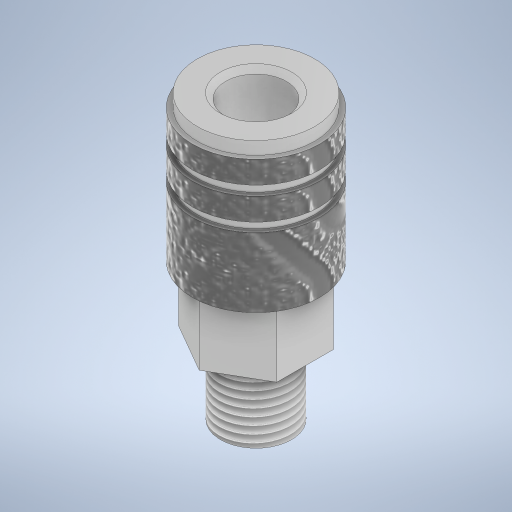
# Autodesk Inventor part: AcopleHembra
Saved by Autodesk Inventor 2024 (Build 280153000, 153)
## iProperties
Created: 2024-04-30
Part Number: AcopleHembra
Material: Genérico
Document SubType Name: Modeling
Designer: alexa
Density: 1 g/cm^3
Appearance: Valor por defecto
Author: alexa
Autodesk Inventor part; units mm, degrees
ref_plane "YZ Plane" through (0, 0, 0) normal (1, 0, 0) x (0, 1, 0)
ref_plane "XZ Plane" through (0, 0, 0) normal (0, 1, 0) x (-1, 0, 0)
ref_plane "XY Plane" through (0, 0, 0) normal (0, 0, 1) x (1, 0, 0)
sketch "Sketch1" plane through (0, 0, 0) normal (0, 1, 0) x (-1, 0, 0)
  circle A0 centre (0, 0) radius 6.65
  dimension "d0" = 13.3
  constraints: 1 centre point, 1 coincident
  measures "d0" diameter of A0
extrude "Extrusion1" add sketch "Sketch1" along normal blind 13.3
sketch "Sketch2" plane through (0, 13.3, 0) normal (0, 1, 0) x (1, 0, 0)
  line L0 (0, 10.65) -> (9.2232, 5.325)
  line L1 (9.2232, 5.325) -> (9.2232, -5.325)
  line L2 (9.2232, -5.325) -> (0, -10.65)
  line L3 (0, -10.65) -> (-9.2232, -5.325)
  line L4 (-9.2232, -5.325) -> (-9.2232, 5.325)
  line L5 (-9.2232, 5.325) -> (0, 10.65)
  point P0 (0, 0)
  point P1 (0, 0)
  constraints: 12 end point, 13 other
extrude "Extrusion2" add sketch "Sketch2" along normal blind 12.4
sketch "Sketch3" plane through (0, 25.7, 0) normal (0, 1, 0) x (1, 0, 0)
  circle A0 centre (0, 0) radius 11.9
  dimension "d6" = 23.8
  constraints: 1 centre point, 1 coincident
  measures "d6" diameter of A0
extrude "Extrusion3" add sketch "Sketch3" along normal blind 13
sketch "Sketch4" plane through (0, 38.7, 0) normal (0, 1, 0) x (1, 0, 0)
  circle A0 centre (0, 0) radius 11
  dimension "d9" = 22
  constraints: 1 centre point, 1 coincident
  measures "d9" diameter of A0
extrude "Extrusion4" add sketch "Sketch4" along normal blind 1.7
sketch "Sketch5" plane through (0, 40.4, 0) normal (0, 1, 0) x (1, 0, 0)
  circle A0 centre (0, 0) radius 11.9
  constraints: 1 centre point, 1 coincident
extrude "Extrusion5" add sketch "Sketch5" along normal blind 4.2
sketch "Sketch6" plane through (0, 44.6, 0) normal (0, 1, 0) x (1, 0, 0)
  circle A0 centre (0, 0) radius 11
  constraints: 1 centre point, 1 coincident
extrude "Extrusion6" add sketch "Sketch6" along normal blind 1.8
sketch "Sketch7" plane through (0, 46.4, 0) normal (0, 1, 0) x (1, 0, 0)
  circle A0 centre (0, 0) radius 11.8989
  constraints: 1 centre point, 1 coincident
extrude "Extrusion7" add sketch "Sketch7" along normal blind 4.2
sketch "Sketch8" plane through (0, 50.6, 0) normal (0, 1, 0) x (1, 0, 0)
  circle A0 centre (0, 0) radius 11
  constraints: 1 centre point, 1 coincident
extrude "Extrusion8" add sketch "Sketch8" along normal blind 2.4
thread "Thread1" size "1/4" designation "1/4 - 18 NPT" standard "NPT" length 15.103
sketch "Sketch9" plane through (0, 53, 0) normal (0, 1, 0) x (1, 0, 0)
  circle A0 centre (0, 0) radius 5.7
  dimension "d22" = 11.4
  constraints: 1 centre point, 1 coincident
  measures "d22" diameter of A0
extrude "Extrusion9" cut sketch "Sketch9" against normal blind 20.6
chamfer "Chamfer1" distance 1 angle 45 1 edges at (-5.7, 53, 0)
sketch "Sketch10" plane through (0, 0, 0) normal (0, -1, 0) x (1, 0, 0)
  circle A0 centre (0, 0) radius 3.75
  dimension "d28" = 7.5
  constraints: 1 centre point, 1 coincident
  measures "d28" diameter of A0
extrude "Extrusion10" cut sketch "Sketch10" against normal blind 29.4
body "Solid1"
